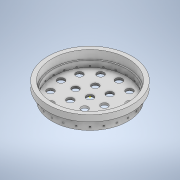
# Autodesk Inventor part: basev_1
Saved by Autodesk Inventor 2022 (Build 260153000, 153)
## iProperties
Created: 2021-07-24
Part Number: basev_1
Material: Generic
Document SubType Name: Modeling
Designer: WASHINGTON
Density: 1 g/cm^3
Appearance: Default
Author: WASHINGTON
Autodesk Inventor part; units mm, degrees
ref_plane "YZ Plane" through (0, 0, 0) normal (1, 0, 0) x (0, 1, 0)
ref_plane "XZ Plane" through (0, 0, 0) normal (0, 1, 0) x (-1, 0, 0)
sketch "Sketch1" plane through (0, 0, 0) normal (0, 1, 0) x (-1, 0, 0)
  circle A0 centre (0, 0) radius 55
  circle A1 centre (0, 0) radius 8 construction
  line L0 (0, 0) -> (21, 0)
  line L1 (0, 0) -> (42, 0)
  circle A2 centre (21, 0) radius 8 construction
  circle A3 centre (42, 0) radius 8 construction
  circle A4 centre (0, 0) radius 5
  circle A5 centre (21, 0) radius 5
  circle A6 centre (42, 0) radius 5
  circle A7 centre (10.5, 18.1865) radius 5
  circle A8 centre (-10.5, 18.1865) radius 5
  circle A9 centre (-21, 0) radius 5
  circle A10 centre (-10.5, -18.1865) radius 5
  circle A11 centre (10.5, -18.1865) radius 5
  circle A12 centre (36.3731, 21) radius 5
  circle A13 centre (21, 36.3731) radius 5
  circle A14 centre (0, 42) radius 5
  circle A15 centre (-21, 36.3731) radius 5
  circle A16 centre (-36.3731, 21) radius 5
  circle A17 centre (-42, 0) radius 5
  circle A18 centre (-36.3731, -21) radius 5
  circle A19 centre (-21, -36.3731) radius 5
  circle A20 centre (0, -42) radius 5
  circle A21 centre (21, -36.3731) radius 5
  circle A22 centre (36.3731, -21) radius 5
  circle A23 centre (0, 0) radius 53
  dimension "d0" = 110
  dimension "d1" = 16
  dimension "d2" = 21
  dimension "d3" = 42
  dimension "d4" = 16
  dimension "d5" = 16
  dimension "d14" = 10
  dimension "d15" = 10
  dimension "d16" = 10
  dimension "d19" = 360
  dimension "d23" = 360
  dimension "d25" = 106
  constraints: 24 centre point, 8 coincident, 4 end point, 1 horizontal, 1 point on line, 38 other
  measures "d0" diameter of A0
  measures "d1" diameter of A1
  measures "d2" distance of L0.start L0.end
  measures "d3" distance of L0.start L1.end
  measures "d4" diameter of A2
  measures "d5" diameter of A3
  measures "d14" diameter of A4
  measures "d15" diameter of A5
  measures "d16" diameter of A6
  measures "d25" diameter of A23
extrude "Extrusion1" add sketch "Sketch1" along normal blind 3 contours A23
extrude "Extrusion3" add sketch "Sketch1" along normal blind 12 contours A0
ref_plane "Work Plane1" through (0, 0, 55) normal (0, 0, 1) x (1, 0, 0)
sketch "Sketch2" plane through (0, 3, 0) normal (0, 1, 0) x (1, 0, 0)
  point P0 (0, 0)
sketch "Sketch3" plane through (0, 0, 55) normal (0, 0, 1) x (1, 0, 0)
  line L0 (0, 0) -> (0, 4.5)
  circle A0 centre (0, 4.5) radius 1
  dimension "d33" = 4.5
  dimension "d34" = 2
  constraints: 2 end point, 1 centre point, 1 coincident, 1 vertical
  measures "d33" distance of L0.start L0.end
  measures "d34" diameter of A0
extrude "Extrusion4" cut sketch "Sketch3" against normal blind 3
pattern_circular "Circular Pattern1" count 24 over 360 about axis through (0, 0, 0) along (0, 1, 0) of "Extrusion4"
sketch "Sketch4" plane through (0, 12, 0) normal (0, 1, 0) x (1, 0, 0)
  circle A0 centre (0, 0) radius 5 projected
  circle A1 centre (0, 0) radius 55
  circle A2 centre (0, 0) radius 56
  dimension "d40" = 112
  constraints: 2 centre point, 2 coincident
  measures "d40" diameter of A2
extrude "Extrusion5" add sketch "Sketch4" along normal blind 3 contours A2
sketch "Sketch5" plane through (0, 15, 0) normal (0, 1, 0) x (1, 0, 0)
  circle A0 centre (0, 0) radius 5 projected
  circle A1 centre (0, 0) radius 55
  circle A2 centre (0, 0) radius 61
  dimension "d43" = 110
  dimension "d44" = 122
  constraints: 2 centre point, 2 coincident
  measures "d43" diameter of A1
  measures "d44" diameter of A2
extrude "Extrusion6" add sketch "Sketch5" along normal blind 9 contours A2
body "Solid1"
